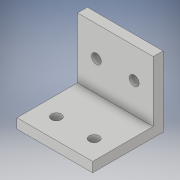
# Autodesk Inventor part: Angle
Saved by Autodesk Inventor 2018 (Build 220112000, 112)
## iProperties
Created: 2017-04-14
Part Number: Angle
Material: Generic
Document SubType Name: Modeling
Designer: Administrator
Density: 1 g/cm^3
Appearance: Default
Author: Administrator
Autodesk Inventor part; units mm, degrees
ref_plane "YZ Plane" through (0, 0, 0) normal (1, 0, 0) x (0, 1, 0)
ref_plane "XZ Plane" through (0, 0, 0) normal (0, 1, 0) x (-1, 0, 0)
ref_plane "XY Plane" through (0, 0, 0) normal (0, 0, 1) x (1, 0, 0)
sketch "Sketch1" plane through (0, 0, 0) normal (0, 0, 1) x (1, 0, 0)
  line L0 (-25, 0) -> (25, 0)
  line L1 (25, 0) -> (25, 46.5)
  line L2 (25, 46.5) -> (-25, 46.5)
  line L3 (-25, 46.5) -> (-25, 0)
  circle A0 centre (-12.5, 26.5) radius 3.25
  circle A1 centre (12.5, 26.5) radius 3.25
  point P0 (0, 0)
  dimension "d0" = 50
  dimension "d1" = 46.5
  dimension "d2" = 6.5
  dimension "d3" = 6.5
  constraints: 8 end point, 2 centre point, 2 parallel, 1 horizontal, 1 perpendicular
  measures "d0" distance of L2.end L1.end
  measures "d1" distance of L1.end L0.end
  measures "d2" diameter of A0
  measures "d3" diameter of A1
extrude "Extrusion1" add sketch "Sketch1" along normal blind 6.5
sketch "Sketch2" plane through (0, 0, 6.5) normal (0, 0, 1) x (1, 0, 0)
  line L0 (-25, 0) -> (25, 0)
  line L1 (25, 0) -> (25, 6.5)
  line L2 (25, 6.5) -> (-25, 6.5)
  line L3 (-25, 6.5) -> (-25, 0)
  point P0 (0, 0)
  dimension "d6" = 50
  dimension "d7" = 6.5
  constraints: 8 end point, 2 parallel, 1 horizontal, 1 perpendicular
  measures "d6" distance of L2.end L1.end
  measures "d7" distance of L1.end L0.end
extrude "Extrusion2" add sketch "Sketch2" along normal blind 40
sketch "Sketch3" plane through (-25, 6.5, 6.5) normal (0, 1, 0) x (1, 0, 0)
  circle A0 centre (12.5, -26.5) radius 3.25
  circle A1 centre (37.5, -26.5) radius 3.25
  point P0 (25, 6.5)
  dimension "d10" = 6.5
  dimension "d11" = 6.5
  constraints: 2 centre point
  measures "d10" diameter of A0
  measures "d11" diameter of A1
hole "Hole1" at (-12.5, 6.5, 33) direction (0, -1, 0) diameter 6.5 end through all
sketch "Sketch4" plane through (-25, 6.5, 6.5) normal (0, 1, 0) x (1, 0, 0)
  circle A0 centre (37.5, -26.5) radius 3.25
  point P0 (25, 6.5)
  dimension "d19" = 6.5
  constraints: 1 centre point
  measures "d19" diameter of A0
hole "Hole2" at (12.5, 6.5, 33) direction (0, -1, 0) diameter 6.5 end through all
body "Solid1"
